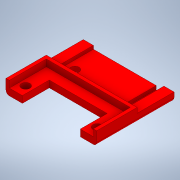
# Autodesk Inventor part: imu_mount
Saved by Autodesk Inventor 2020 (Build 240168000, 168)
## iProperties
Created: 2019-12-07
Part Number: imu_mount
Material: Generic
Document SubType Name: Modeling
Designer: ZEUSLAP
Density: 1 g/cm^3
Appearance: Default
Author: ZEUSLAP
Autodesk Inventor part; units mm, degrees
ref_plane "YZ Plane" through (0, 0, 0) normal (1, 0, 0) x (0, 1, 0)
ref_plane "XZ Plane" through (0, 0, 0) normal (0, 1, 0) x (-1, 0, 0)
ref_plane "XY Plane" through (0, 0, 0) normal (0, 0, 1) x (1, 0, 0)
sketch "Sketch1" plane through (0, 0, 0) normal (0, 0, 1) x (1, 0, 0)
  line L0 (-13.5, 6) -> (13.5, 6)
  line L1 (13.5, 6) -> (13.5, -6)
  line L2 (13.5, -6) -> (-13.5, -6)
  line L3 (-13.5, -6) -> (-13.5, 6)
  line L4 (-8.625, -6) -> (-8.625, 2)
  line L5 (-8.625, 2) -> (8.625, 2)
  line L6 (8.625, 2) -> (8.625, -6)
  line L7 (0, 19.1515) -> (0, -21.0963) construction
  line L8 (-12.5, -6) -> (-12.5, 5)
  line L9 (-12.5, 5) -> (12.5, 5)
  line L10 (12.5, 5) -> (12.5, -6)
  circle A0 centre (10.625, -3) radius 1.25
  circle A1 centre (-10.625, -3) radius 1.25
  line L11 (10.625, -5.3094) -> (8.625, -4.1547)
  line L12 (8.625, -4.1547) -> (8.625, -1.8453)
  line L13 (8.625, -1.8453) -> (10.625, -0.6906)
  line L14 (10.625, -0.6906) -> (12.625, -1.8453)
  line L15 (12.625, -1.8453) -> (12.625, -4.1547)
  line L16 (12.625, -4.1547) -> (10.625, -5.3094)
  line L17 (-10.625, -5.3094) -> (-12.625, -4.1547)
  line L18 (-12.625, -4.1547) -> (-12.625, -1.8453)
  line L19 (-12.625, -1.8453) -> (-10.625, -0.6906)
  line L20 (-10.625, -0.6906) -> (-8.625, -1.8453)
  line L21 (-8.625, -1.8453) -> (-8.625, -4.1547)
  line L22 (-8.625, -4.1547) -> (-10.625, -5.3094)
  line L23 (13.5, 6) -> (13.5, 17)
  line L24 (13.5, 17) -> (-13.5, 17)
  line L25 (-13.5, 17) -> (-13.5, 6)
  point P0 (0, 0)
  point P1 (-13.5, 0)
  point P2 (0, 6)
  point P3 (0, 16)
  dimension "d2" = 17.25
  dimension "d3" = 1
  dimension "d4" = 1
  dimension "d5" = 3
  dimension "d10" = 2.5
  dimension "d11" = 21.25
  dimension "d12" = 8
  dimension "d13" = 2
  dimension "d16" = 11
  dimension "d17" = 25
  dimension "d19" = 15
  constraints: 52 end point, 6 perpendicular, 5 point on line, 4 vertical, 2 centre point, 2 coincident, 2 horizontal, 2 midpoint, 2 parallel, 2 vertical alignment, 1 collinear, 1 equal radius, 1 horizontal alignment, 30 other
  measures "d2" distance of L4.end L5.end
  measures "d3" distance between parallel lines of L1 L10
  measures "d4" distance between parallel lines of L0 L9
  measures "d5" distance between parallel lines of L9 L5
  measures "d10" diameter of A1
  measures "d11" distance of A1.centre A0.centre
  measures "d12" distance from line of L9 A0.centre
  measures "d13" distance from line of L12 A0.centre
  measures "d16" distance of L8.start L8.end
  measures "d17" distance of L8.end L9.end
  measures "d19" distance between parallel lines of L24 L5
extrude "body" add sketch "Sketch1" along normal blind 2 contours L0 L1 L2 L10 L16 L15 L14 L9 L8 L19 L18 L17 L3 | L8 L17 L22 L4 L2 | L2 L6 L11 L16 L10 | L17 L18 L19 L8 | L8 L19 L20 L4 L22 L17 | L16 L11 L6 L13 L14 L10 | L10 L14 L15 L16 | L8 L9 L10 L14 L13 L6 L5 L4 L20 L19
extrude "borders" add sketch "Sketch1" along normal blind 4 contours L0 L1 L2 L10 L16 L15 L14 L9 L8 L19 L18 L17 L3 | L17 L18 L19 L8 | L10 L14 L15 L16
extrude "nut_recesses" [suppressed]
extrude "jut out for imu" add sketch "Sketch1" along normal blind 2.5 contours L25 L24 L23 L0
sketch "Sketch2" plane through (0, 0, 2.5) normal (0, 0, 1) x (1, 0, 0)
  line L0 (-10.5, 20) -> (10.5, 20)
  line L1 (10.5, 20) -> (10.5, 6.5)
  line L2 (10.5, 6.5) -> (-10.5, 6.5)
  line L3 (-10.5, 6.5) -> (-10.5, 20)
  circle A0 centre (-8, 9) radius 1.25
  line L4 (13.5, 6) -> (-13.5, 6) projected
  line L5 (10.23, 6.5) -> (10.23, 20)
  line L6 (8.23, 20) -> (8.23, 6.5)
  line L7 (8.23, 13.25) -> (10.23, 13.25) construction
  point P0 (0, 0)
  point P1 (0, 20)
  point P2 (9.23, 13.25)
  dimension "d32" = 21
  dimension "d33" = 13.5
  dimension "d34" = 2.5
  dimension "d35" = 2.5
  dimension "d36" = 2.5
  dimension "d44" = 0.5
  dimension "d45" = 2
  dimension "d46" = 1.27
  constraints: 14 end point, 4 midpoint, 4 point on line, 3 perpendicular, 2 parallel, 1 centre point, 1 horizontal, 1 vertical alignment
  measures "d32" distance of L0.start L0.end
  measures "d33" distance of L0.end L1.end
  measures "d34" distance from line of L3 A0.centre
  measures "d35" distance from line of L2 A0.centre
  measures "d36" diameter of A0
  measures "d44" distance between parallel lines of L4 L2
  measures "d45" distance between parallel lines of L5 L6
  measures "d46" distance from line of L1 point (9.23, 13.25)
extrude "recess for imu" cut sketch "Sketch2" along normal blind 10 and the other way blind 1 contours L0 L6 L2 L3 | L0 L5 L2 L6 | L0 L1 L2 L5 | A0
extrude "hole for imu" cut sketch "Sketch2" against normal blind 10 contours A0
fillet "Fillet2" radius 1 3 edges at (-13.5, 5.5, 0) (0, 17, 0) (13.5, 5.5, 0)
extrude "Extrusion9" cut sketch "Sketch2" against normal blind 2 contours L0 L5 L2 L6
equation "\"d4\" = d3"
body "Solid1"
